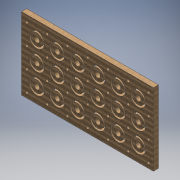
# Autodesk Inventor part: BearingSiliconeMold_2
Saved by Autodesk Inventor 2016 (Build 200138000, 138)
## iProperties
Created: 2015-12-06
Part Number: BearingSiliconeMold_2
Material: MDF Medium Density Fiberboard
Document SubType Name: Modeling
Designer: DonMo
Density: 0.8 g/cm^3
Appearance: Cardboard - Corrugated
Author: DonMo
Autodesk Inventor part; units mm, degrees
ref_plane "YZ Plane" through (0, 0, 0) normal (1, 0, 0) x (0, 1, 0)
ref_plane "XZ Plane" through (0, 0, 0) normal (0, 1, 0) x (-1, 0, 0)
ref_plane "XY Plane" through (0, 0, 0) normal (0, 0, 1) x (1, 0, 0)
sketch "Sketch1" plane through (0, 0, 0) normal (0, 1, 0) x (-1, 0, 0)
  circle A0 centre (0, 0) radius 9
  circle A1 centre (0, 0) radius 7
  circle A2 centre (12, -12) radius 1.715
  line L0 (0, 0) -> (0, -7) construction
  line L1 (0, 0) -> (9, 0) construction
  circle A3 centre (0, 0) radius 3.175
  line L2 (18, -66) -> (-138, -66)
  line L3 (-138, -66) -> (-138, 19.715)
  line L4 (-138, 19.715) -> (18, 19.715)
  line L5 (18, 19.715) -> (18, -66)
  circle A4 centre (12, 12) radius 1.715
  circle A5 centre (-12, 12) radius 1.715
  circle A6 centre (-12, -12) radius 1.715
  line L6 (12, -12) -> (0, 0) construction
  circle A7 centre (0, -24) radius 9
  circle A8 centre (0, -24) radius 7
  circle A9 centre (0, -24) radius 3.175
  circle A10 centre (12, -36) radius 1.715
  circle A11 centre (-12, -36) radius 1.715
  circle A12 centre (0, -48) radius 9
  circle A13 centre (0, -48) radius 7
  circle A14 centre (0, -48) radius 3.175
  circle A15 centre (12, -60) radius 1.715
  circle A16 centre (-12, -60) radius 1.715
  circle A17 centre (-36, 12) radius 1.715
  circle A18 centre (-24, 0) radius 9
  circle A19 centre (-24, 0) radius 7
  circle A20 centre (-24, 0) radius 3.175
  circle A21 centre (-36, -12) radius 1.715
  circle A22 centre (-24, -24) radius 9
  circle A23 centre (-24, -24) radius 7
  circle A24 centre (-24, -24) radius 3.175
  circle A25 centre (-36, -36) radius 1.715
  circle A26 centre (-24, -48) radius 9
  circle A27 centre (-24, -48) radius 7
  circle A28 centre (-24, -48) radius 3.175
  circle A29 centre (-36, -60) radius 1.715
  circle A30 centre (-60, 12) radius 1.715
  circle A31 centre (-48, 0) radius 9
  circle A32 centre (-48, 0) radius 7
  circle A33 centre (-48, 0) radius 3.175
  circle A34 centre (-60, -12) radius 1.715
  circle A35 centre (-48, -24) radius 9
  circle A36 centre (-48, -24) radius 7
  circle A37 centre (-48, -24) radius 3.175
  circle A38 centre (-60, -36) radius 1.715
  circle A39 centre (-48, -48) radius 9
  circle A40 centre (-48, -48) radius 7
  circle A41 centre (-48, -48) radius 3.175
  circle A42 centre (-60, -60) radius 1.715
  circle A43 centre (-84, 12) radius 1.715
  circle A44 centre (-72, 0) radius 9
  circle A45 centre (-72, 0) radius 7
  circle A46 centre (-72, 0) radius 3.175
  circle A47 centre (-84, -12) radius 1.715
  circle A48 centre (-72, -24) radius 9
  circle A49 centre (-72, -24) radius 7
  circle A50 centre (-72, -24) radius 3.175
  circle A51 centre (-84, -36) radius 1.715
  circle A52 centre (-72, -48) radius 9
  circle A53 centre (-72, -48) radius 7
  circle A54 centre (-72, -48) radius 3.175
  circle A55 centre (-84, -60) radius 1.715
  circle A56 centre (-108, 12) radius 1.715
  circle A57 centre (-96, 0) radius 9
  circle A58 centre (-96, 0) radius 7
  circle A59 centre (-96, 0) radius 3.175
  circle A60 centre (-108, -12) radius 1.715
  circle A61 centre (-96, -24) radius 9
  circle A62 centre (-96, -24) radius 7
  circle A63 centre (-96, -24) radius 3.175
  circle A64 centre (-108, -36) radius 1.715
  circle A65 centre (-96, -48) radius 9
  circle A66 centre (-96, -48) radius 7
  circle A67 centre (-96, -48) radius 3.175
  circle A68 centre (-108, -60) radius 1.715
  circle A69 centre (-132, 12) radius 1.715
  circle A70 centre (-120, 0) radius 9
  circle A71 centre (-120, 0) radius 7
  circle A72 centre (-120, 0) radius 3.175
  circle A73 centre (-132, -12) radius 1.715
  circle A74 centre (-120, -24) radius 9
  circle A75 centre (-120, -24) radius 7
  circle A76 centre (-120, -24) radius 3.175
  circle A77 centre (-132, -36) radius 1.715
  circle A78 centre (-120, -48) radius 9
  circle A79 centre (-120, -48) radius 7
  circle A80 centre (-120, -48) radius 3.175
  circle A81 centre (-132, -60) radius 1.715
  point P0 (9, -24)
  point P1 (0, -31)
  point P2 (9, -48)
  point P3 (0, -55)
  point P4 (-15, 0)
  point P5 (-24, -7)
  point P6 (-15, -24)
  point P7 (-24, -31)
  point P8 (-15, -48)
  point P9 (-24, -55)
  point P10 (-39, 0)
  point P11 (-48, -7)
  point P12 (-39, -24)
  point P13 (-48, -31)
  point P14 (-39, -48)
  point P15 (-48, -55)
  point P16 (-63, 0)
  point P17 (-72, -7)
  point P18 (-63, -24)
  point P19 (-72, -31)
  point P20 (-63, -48)
  point P21 (-72, -55)
  point P22 (-87, 0)
  point P23 (-96, -7)
  point P24 (-87, -24)
  point P25 (-96, -31)
  point P26 (-87, -48)
  point P27 (-96, -55)
  point P28 (-111, 0)
  point P29 (-120, -7)
  point P30 (-111, -24)
  point P31 (-120, -31)
  point P32 (-111, -48)
  point P33 (-120, -55)
  dimension "d0" = 18
  dimension "d1" = 2
  dimension "d2" = 3.43
  dimension "d6" = 6.35
  dimension "d27" = 360
  dimension "d29" = 45
  dimension "d30" = 12
  dimension "d33" = 24
  dimension "d40" = 24
  dimension "d45" = 6
  dimension "d46" = 6
  dimension "d47" = 6
  dimension "d48" = 6
  constraints: 46 centre point, 37 coincident, 33 horizontal, 18 horizontal alignment, 18 vertical alignment, 14 end point, 6 vertical, 2 parallel, 1 perpendicular, 231 other
  measures "d2" diameter of A2
  measures "d6" diameter of A3
  measures "d29" angle of L0 L6
  measures "d30" horizontal distance of L6.start point (0, 0)
  measures "d33" distance of point (0, 0) point (0, -24)
  measures "d40" distance of A5.centre A17.centre
  measures "d45" distance edge to line of A4 L4
  measures "d46" distance from line of L5 A4.centre
  measures "d47" distance from line of L2 A15.centre
  measures "d48" distance from line of L3 A69.centre
extrude "Extrusion3" add sketch "Sketch1" along normal blind 5.95
equation "\"d0\" = 0.75 * BearingDiameter"
equation "\"d1\" = SiliconeOverlapThickness"
equation "\"d2\" = HoldScrewDiameter"
equation "\"d6\" = DowlDiameter"
equation "\"d49\" = WoodThickness"
equation "\"BearingDiameter\" = 24"
equation "\"SiliconeOverlapThickness\" = 2"
equation "\"HoldScrewDiameter\" = 3.43"
equation "\"DowlDiameter\" = 6.35"
equation "\"WoodThickness\" = 5.95"
body "Solid3"
